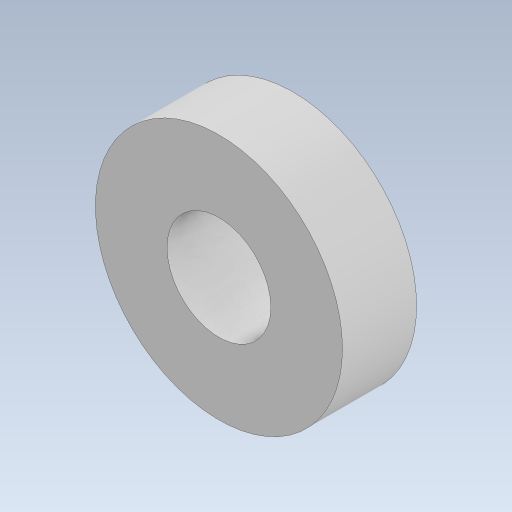
# Autodesk Inventor part: 零件14
Saved by Autodesk Inventor 2023 (Build 270158000, 158)
## iProperties
Created: 2023-04-16
Part Number: 零件14
Material: 一般
Document SubType Name: Modeling
Designer: JOU
Density: 1 g/cm^3
Appearance: 預設
Author: JOU
Autodesk Inventor part; units mm, degrees
ref_plane "YZ Plane" through (0, 0, 0) normal (1, 0, 0) x (0, 1, 0)
ref_plane "XZ Plane" through (0, 0, 0) normal (0, 1, 0) x (-1, 0, 0)
ref_plane "XY Plane" through (0, 0, 0) normal (0, 0, 1) x (1, 0, 0)
sketch "草圖4" plane through (0, 0, 0) normal (0, 0, 1) x (1, 0, 0)
  circle A0 centre (0, 0) radius 2.1
  circle A1 centre (0, 0) radius 5
  dimension "d24" = 4.2
  dimension "d25" = 10
  constraints: 2 centre point, 2 coincident
  measures "d24" diameter of A0
  measures "d25" diameter of A1
extrude "擠出3" add sketch "草圖4" along normal blind 3
